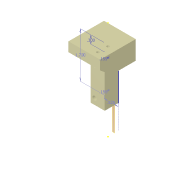
# Autodesk Inventor part: Lower Lift Limit & Stop
Saved by Autodesk Inventor 2018 (Build 220112000, 112)
## iProperties
Created: 2018-12-24
Part Number: Lower Lift Limit & Stop
Material: Generic
Document SubType Name: Modeling
Designer: ball
Density: 1 g/cm^3
Appearance: Default
Author: ball
Autodesk Inventor part; units mm, degrees
ref_plane "YZ Plane" through (0, 0, 0) normal (1, 0, 0) x (0, 1, 0)
ref_plane "XZ Plane" through (0, 0, 0) normal (0, 1, 0) x (-1, 0, 0)
ref_plane "XY Plane" through (0, 0, 0) normal (0, 0, 1) x (1, 0, 0)
ref_plane "Work Plane1" through (0, 0, 0) normal (0, 0, 1) x (1, 0, 0)
sketch "Sketch1" plane through (0, 0, 0) normal (0, 0, 1) x (1, 0, 0)
  line L0 (9.525, 9.7566) -> (9.525, 85.9566) construction
  line L1 (-3.1132, 67.9011) -> (3.1132, 67.9011) construction
  line L2 (-3.1132, 34.8811) -> (3.1132, 34.8811) construction
  line L3 (9.525, 75.5211) -> (-9.525, 75.5211) construction
  line L4 (9.525, 75.5211) -> (-3.81, 75.5211) construction
  line L5 (-3.81, 75.5211) -> (-3.81, 32.3411) construction
  line L6 (-3.81, 32.3411) -> (9.525, 32.3411) construction
  line L7 (9.525, 75.5211) -> (-3.81, 75.5211)
  line L8 (-3.81, 75.5211) -> (-3.81, 32.3411)
  line L9 (-3.81, 32.3411) -> (9.525, 32.3411)
  arc A0 (1.7468, 65.0042) -> (1.3298, 63.7199) centre (0, 64.8615) ccw construction
  arc A1 (1.7468, 38.0634) -> (1.3298, 36.7792) centre (0, 37.9208) ccw construction
  circle A2 centre (0, 64.8615) radius 1.9685
  circle A3 centre (0, 37.9208) radius 1.9685
  line L10 (9.525, 32.3411) -> (9.525, 75.5211)
  point P0 (0, 0)
  dimension "d0" = 7.62
  dimension "d1" = 13.335
  dimension "d2" = 43.18
  dimension "d6" = 3.937
  dimension "d7" = 3.937
  constraints: 22 end point, 4 centre point, 4 horizontal, 4 point on circle, 2 coincident, 2 parallel, 2 perpendicular, 1 collinear, 1 point on line, 1 vertical, 14 other
  measures "d0" distance between parallel lines of L3 L1
  measures "d1" distance of L6.end L5.end
  measures "d2" distance of L5.end L4.end
  measures "d6" diameter of A2
  measures "d7" diameter of A3
extrude "Extrusion1" add sketch "Sketch1" along normal blind 12.7 contours L10 L9 L8 L7 | A2 | A3
extrude "Extrusion2" cut sketch "Sketch1" along normal blind 12.7 contours A2 | A3
ref_plane "Work Plane2" through (0, 0, 0) normal (0, 0, 1) x (1, 0, 0)
sketch "Sketch2" plane through (0, 0, 0) normal (0, 0, 1) x (1, 0, 0)
  line L0 (-3.81, 75.5211) -> (9.525, 75.5211) projected
  line L1 (-3.81, 75.5211) -> (12.7, 75.5211) construction
  line L2 (-3.81, 75.5211) -> (26.289, 75.5211)
  line L3 (26.289, 75.5211) -> (26.289, 93.3011)
  line L4 (26.289, 93.3011) -> (-3.81, 93.3011)
  line L5 (-3.81, 93.3011) -> (-3.81, 75.5211)
  point P0 (0, 0)
  dimension "d10" = 30.099
  dimension "d11" = 17.78
  constraints: 10 end point, 2 parallel, 1 collinear, 1 horizontal, 1 perpendicular
  measures "d10" distance of L4.end L3.end
  measures "d11" distance between parallel lines of L4 L2
extrude "Extrusion3" add sketch "Sketch2" along normal blind 33.782
sketch "Sketch3" plane through (-3.81, 93.3011, 0) normal (0, 1, 0) x (1, 0, 0)
  point P0 (3.81, 0)
fillet "Fillet1" radius 3.175 1 edges at (2.8575, 75.5211, 12.7)
sketch "Sketch5" plane through (-3.81, 93.3011, 0) normal (0, 1, 0) x (1, 0, 0)
  circle A0 centre (22.987, -28.6004) radius 1.1938 construction
  line L0 (30.099, -33.782) -> (0, -33.782) construction
  line L1 (30.099, 0) -> (30.099, -33.782) construction
  circle A1 centre (22.987, -19.0754) radius 1.1938 construction
  point P0 (3.81, 0)
  dimension "d22" = 2.3876
  dimension "d23" = 5.1816
  dimension "d24" = 7.112
  dimension "d25" = 2.3876
  dimension "d26" = 9.525
  constraints: 2 centre point
  measures "d22" diameter of A0
  measures "d23" distance from line of L0 A0.centre
  measures "d24" distance from line of L1 A0.centre
  measures "d25" diameter of A1
  measures "d26" distance of A1.centre A0.centre
hole "Hole2" at (19.177, 93.3011, 28.6004) at (19.177, 93.3011, 19.0754) direction (0, -1, 0) diameter 2.3876 depth 12.7
sketch "Sketch6" plane through (26.289, 75.5211, 0) normal (1, 0, 0) x (0, 0, -1)
  line L0 (0, 17.78) -> (-33.782, 17.78) projected
  line L1 (-33.782, 0) -> (-33.782, 17.78) projected
  line L2 (0, 0) -> (-33.782, 0) projected
  line L3 (0, 0) -> (0, 17.78) projected
  line L4 (-15.875, 0) -> (-33.782, 0) projected
  line L5 (-22.86, 0) -> (-33.782, 0)
  line L6 (-33.782, 0) -> (-33.782, 8.89)
  line L7 (-22.86, 0) -> (-33.782, 8.89)
  point P0 (0, -75.5211)
  dimension "d36" = 22.86
  dimension "d37" = 8.89
  constraints: 6 end point, 1 collinear, 1 midpoint, 1 point on line
  measures "d36" distance from line of L3 L5.start
  measures "d37" distance from line of L0 L6.end
extrude "Extrusion4" cut sketch "Sketch6" against normal through all contours L7 L2 L1
body "Solid1"
